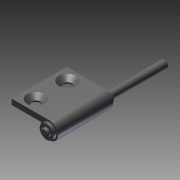
# Autodesk Inventor part: HHPFRN5-1
Saved by Autodesk Inventor 2015 SP1 (Build 190203100, 203)
## iProperties
Category: PARTsolutions
Company: MISUMI
Created: 2015-01-26
Part Number: HHPFRN5-1
Catalog Web Link: www.cadenas.de
Description: HHPFLN, HHPFRN-1-Aluminum Flag Hinges
Vendor: MISUMI
Document SubType Name: Modeling
Designer: PARTuser1
Manufacturer: MISUMI
Mass: 6.43029 g
Surface Area: 36.1077 cm^2
Volume: 6.43029 cm^3
Density: 1 g/cm^3
Material: Generic
Appearance: PSOLRGB-192-192-192
PSOL_IDENT_0: {\\10.0.0.236\data_v8\23d-libs\misumi\metric\39_accessories_for_al_extrusions\hhpfln_1.prj},177 {VTY
PSOL_IDENT_1: P=3D},{NB=HHPFRN5-1},{LINA=HHPFRN5-1},{NN=HHPFLN, HHPFRN-1},{DATE=17.11.2014 05:31:02},{GEOMDATE=07.
PSOL_IDENT_2: 05.2009 08:35:00},{VERSION=},{LINEID=10},{LINESUBID=-1},{WBVAR=TS,ALT1}  {NB=HHPFRN5-1},{LINA=HHPFRN
PSOL_IDENT_3: 5-1},{KT=DUMMY},{PN=HHPFRN5},{TYPE=HHPFRN},{TS=HHPFRN},{MAT=6063 Aluminum Bushing - Polyacetal},{ST=
PSOL_IDENT_4: Anodizing},{NO=5},{ALKG=10},{ALN=98},{MASS=36},{L=35},{W=48},{K=7.5},{P=20},{J=8.0},{F=16.0},{V=10.5
PSOL_IDENT_5: },{ND=5.5},{NC=11},{T=3.5},{Y=38.5},{AB=FB5-8},{QB=4},{AN=HNTT5-5},{QN=4},{ALT1=},{NMAT=316 Stainles
PSOL_IDENT_6: s Steel (or Equivalent)},{BMAT=SHFB},{BD=5},{BL=8},{NS=5},{NM=5}
SUPPLIER: MISUMI
ARTICLENO: HHPFRN5-1
BOMINFO: HHPFRN5-1
CREATOR: CADENAS GmbH
Title: HHPFRN5-1
Author: Cadenas PARTsolutions
Comments: Aluminum Flag Hinges
Autodesk Inventor part; units mm, degrees
sketch "Sketch_1" plane through (0, 0, 0) normal (0, 0, 1) x (1, 0, 0)
  line L0 (0, -39.9) -> (0, 36.8)
  line L1 (0, 36.8) -> (2, 36.8)
  line L2 (2, 36.8) -> (2.5, 36.3)
  line L3 (2.5, 36.3) -> (2.5, 0)
  line L4 (2.5, 0) -> (4.4, 0)
  line L5 (4.4, 0) -> (4.4, -0.85)
  line L6 (4.4, -0.85) -> (4.5, -0.85)
  line L7 (4.5, -0.85) -> (4.5, -1.7)
  line L8 (4.5, -1.7) -> (5.5, -1.7)
  line L9 (5.5, -1.7) -> (5.5, -36.7)
  line L10 (5.5, -36.7) -> (4.5, -36.7)
  line L11 (4.5, -36.7) -> (4.5, -37.55)
  line L12 (4.5, -37.55) -> (4.4, -37.55)
  line L13 (4.4, -37.55) -> (4.4, -38.4)
  line L14 (4.4, -38.4) -> (2.5, -38.4)
  line L15 (2.5, -38.4) -> (2.5, -39.4)
  line L16 (2.5, -39.4) -> (2, -39.9)
  line L17 (2, -39.9) -> (0, -39.9)
  line L18 (0, -39.9) -> (0, 36.8)
  constraints: 38 end point
revolve "Revolution1" add sketch "Sketch_1" angle 360 about axis through (0, -39.9, 0) along (0, -1, 0)
sketch "Sketch_3" plane through (0, 0, 5.5) normal (0, 0, 1) x (1, 0, 0)
  line L0 (-24, -1.7) -> (-24, -36.7)
  line L1 (-24, -36.7) -> (0, -36.7)
  line L2 (0, -36.7) -> (0, -1.7)
  line L3 (0, -1.7) -> (-24, -1.7)
  constraints: 8 end point
extrude "Extrusion1" add sketch "Sketch_3" against normal blind 3.5
sketch "Sketch_6" plane through (-16, 0, 0) normal (1, 0, 0) x (0, 0, -1)
  line L0 (-5.5, -9.2) -> (-2, -9.2)
  line L1 (-2, -9.2) -> (-2, -11.95)
  line L2 (-2, -11.95) -> (-2.75, -11.95)
  line L3 (-2.75, -11.95) -> (-5.5, -14.7)
  line L4 (-5.5, -14.7) -> (-5.5, -9.2)
  line L5 (-5.5, -9.2) -> (-2, -9.2)
  constraints: 12 end point
revolve "Revolution2" cut sketch "Sketch_6" angle 360 about axis through (-16, -9.2, 5.5) along (0, 0, 1)
sketch "Sketch_7" plane through (-16, 0, 0) normal (1, 0, 0) x (0, 0, -1)
  line L0 (-5.5, -29.2) -> (-2, -29.2)
  line L1 (-2, -29.2) -> (-2, -31.95)
  line L2 (-2, -31.95) -> (-2.75, -31.95)
  line L3 (-2.75, -31.95) -> (-5.5, -34.7)
  line L4 (-5.5, -34.7) -> (-5.5, -29.2)
  line L5 (-5.5, -29.2) -> (-2, -29.2)
  constraints: 12 end point
revolve "Revolution3" cut sketch "Sketch_7" angle 360 about axis through (-16, -29.2, 5.5) along (0, 0, 1)
ref_plane "1_XY" through (0, 0, 0) normal (0, 1, 0) x (1, 0, 0)
ref_plane "1_YZ" through (0, 0, 0) normal (1, 0, 0) x (0, 0, -1)
ref_plane "1_ZX" through (0, 0, 0) normal (0, 0, -1) x (0, 1, 0)
ref_plane "to_bolt1_XY" through (16, -9.2, 5.5) normal (0, 0, 1) x (1, 0, 0)
ref_plane "to_bolt1_YZ" through (16, -9.2, 5.5) normal (1, 0, 0) x (0, 1, 0)
ref_plane "to_bolt1_ZX" through (16, -9.2, 5.5) normal (0, 1, 0) x (0, 0, 1)
ref_plane "to_bolt2_XY" through (16, -29.2, 5.5) normal (0, 0, 1) x (1, 0, 0)
ref_plane "to_bolt2_YZ" through (16, -29.2, 5.5) normal (1, 0, 0) x (0, 1, 0)
ref_plane "to_bolt2_ZX" through (16, -29.2, 5.5) normal (0, 1, 0) x (0, 0, 1)
ref_plane "to_bolt1_r_XY" through (-16, -9.2, 5.5) normal (0, 0, 1) x (1, 0, 0)
ref_plane "to_bolt1_r_YZ" through (-16, -9.2, 5.5) normal (1, 0, 0) x (0, 1, 0)
ref_plane "to_bolt1_r_ZX" through (-16, -9.2, 5.5) normal (0, 1, 0) x (0, 0, 1)
ref_plane "to_bolt2_r_XY" through (-16, -29.2, 5.5) normal (0, 0, 1) x (1, 0, 0)
ref_plane "to_bolt2_r_YZ" through (-16, -29.2, 5.5) normal (1, 0, 0) x (0, 1, 0)
ref_plane "to_bolt2_r_ZX" through (-16, -29.2, 5.5) normal (0, 1, 0) x (0, 0, 1)
body "Solid1"
